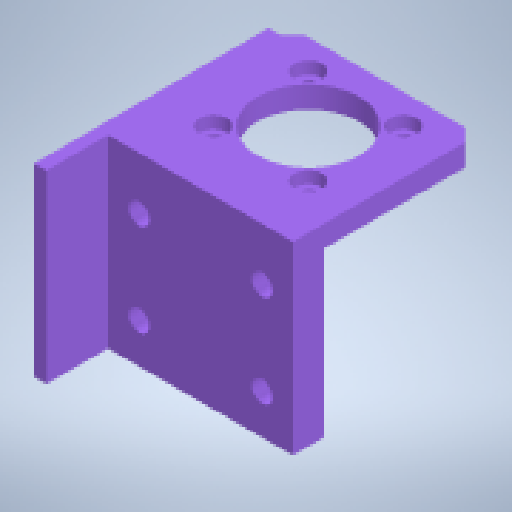
# Autodesk Inventor part: support nema8
Saved by Autodesk Inventor 2025.1 (Build 291241000, 241)
## iProperties
Created: 2025-03-24
Part Number: support nema8
Material: Générique
Document SubType Name: Modeling
Designer: felix
Density: 1 g/cm^3
Appearance: Violet
Author: felix
Autodesk Inventor part; units mm, degrees
ref_plane "YZ Plane" through (0, 0, 0) normal (1, 0, 0) x (0, 1, 0)
ref_plane "XZ Plane" through (0, 0, 0) normal (0, 1, 0) x (-1, 0, 0)
ref_plane "XY Plane" through (0, 0, 0) normal (0, 0, 1) x (1, 0, 0)
sketch "Esquisse1" plane through (0, 0, 0) normal (0, 1, 0) x (-1, 0, 0)
  line L0 (0, 0) -> (30, 0)
  line L1 (30, 0) -> (30, -23)
  line L2 (28, -25) -> (2, -25)
  line L3 (0, -23) -> (0, 0)
  circle A0 centre (15, -12.5) radius 8.25
  line L4 (30, -23) -> (28, -25)
  line L5 (2, -25) -> (0, -23)
  point P0 (0, 0)
  point P1 (30, -25)
  point P2 (0, -25)
  point P3 (11.5, 0)
  point P4 (30, -4)
  point P5 (21, 0)
  point P6 (0, -2)
  point P7 (2, 0)
  dimension "d0" = 25
  dimension "d1" = 30
  dimension "d2" = 16.5
  dimension "d3" = 15
  dimension "d11" = 2
  dimension "d12" = 2
  dimension "d13" = 2
  dimension "d14" = 2
  dimension "d47" = 12.5
  constraints: 13 point on line, 12 end point, 2 parallel, 1 centre point, 1 horizontal, 1 perpendicular
  measures "d0" distance of point (30, 0) point (30, -25)
  measures "d1" distance of point (30, -25) point (0, -25)
  measures "d2" diameter of A0
  measures "d3" distance from line of L3 A0.centre
  measures "d11" distance of L1.end point (30, -25)
  measures "d12" distance of L2.start point (30, -25)
  measures "d13" distance of L2.end point (0, -25)
  measures "d14" distance of L3.start point (0, -25)
  measures "d47" distance from line of L0 A0.centre
extrude "Extrusion1" add sketch "Esquisse1" along normal blind 3.5
sketch "Esquisse2" plane through (0, 3.5, 0) normal (0, 1, 0) x (1, 0, 0)
  circle A0 centre (-15, 12.5) radius 8.25 construction
  circle A1 centre (-15, 12.5) radius 10.8894 construction
  line L0 (-22.7, 4.8) -> (-22.7, 20.2) construction
  line L1 (-22.7, 20.2) -> (-7.3, 20.2) construction
  line L2 (-7.3, 20.2) -> (-7.3, 4.8) construction
  line L3 (-7.3, 4.8) -> (-22.7, 4.8) construction
  point P0 (0, 0)
  dimension "d19" = 15.4
  dimension "d20" = 15.4
  constraints: 8 end point, 5 coincident, 3 point on circle, 2 parallel, 1 centre point, 1 perpendicular, 1 vertical
  measures "d19" distance of L0.start L0.end
  measures "d20" distance of L0.end L1.end
hole "Perçage1" at (-22.7, 3.5, -4.8) at (-22.7, 3.5, -20.2) at (-7.3, 3.5, -20.2) at (-7.3, 3.5, -4.8) direction (0, -1, 0) diameter 2.4 end through all counterbore diameter 4.4 counterbore depth 2 clearance for "Vis d'assemblage à six pans creux" size "M2" standard "Profil M métrique ANSI"
sketch "Esquisse3" plane through (-30, 0, 0) normal (0, 0, 1) x (1, 0, 0)
  line L0 (0, 3.5) -> (30, 3.5) projected
  line L1 (0, 3.5) -> (30, 3.5)
  line L2 (30, 3.5) -> (30, -26.5)
  line L3 (30, -26.5) -> (0, -26.5)
  line L4 (0, -26.5) -> (0, 3.5)
  point P0 (30, 0)
  point P1 (30, 3.5)
  dimension "d29" = 30
  dimension "d48" = 30
  dimension "d49" = 30
  constraints: 8 end point, 2 parallel, 1 horizontal, 1 perpendicular
  measures "d29" distance of L3.end L0.start
  measures "d48" distance of L2.end L3.end
  measures "d49" distance of L0.start L0.end
extrude "Extrusion2" add sketch "Esquisse3" along normal blind 5
sketch "Esquisse4" plane through (-30, 0, -23) normal (-1, 0, 0) x (0, 0, 1)
  line L0 (0, 3.5) -> (28, 3.5) projected
  line L1 (28, 3.5) -> (0, 3.5)
  line L2 (0, 3.5) -> (0, 0)
  line L3 (0, 0) -> (-2, 0) projected
  line L4 (26.5, -26.5) -> (0, 0)
  line L5 (28, 3.5) -> (28, -26.5) projected
  line L6 (28, -26.5) -> (26.5, -26.5)
  line L7 (28, 3.5) -> (38, 3.5)
  line L8 (38, 3.5) -> (38, -26.5)
  line L9 (38, -26.5) -> (21.647, -26.5)
  point P0 (23, 0)
  point P1 (24.5, -21)
  point P2 (0, 3.5)
  point P3 (21, -21)
  dimension "d50" = 30
  dimension "d51" = 30
  dimension "d52" = 10
  constraints: 14 end point, 3 horizontal, 2 perpendicular, 2 point on line, 1 parallel, 1 other
  measures "d50" distance of L0.end L6.start
  measures "d51" distance of L7.end L8.end
  measures "d52" distance of L0.end L7.end
extrude "Extrusion3" add sketch "Esquisse4" along normal blind 2
sketch "Esquisse5" plane through (-30, 0, 0) normal (0, 0, -1) x (-1, 0, 0)
  line L0 (-5, -5) -> (-25, -5) construction
  line L1 (-25, -5) -> (-25, -20) construction
  line L2 (-25, -20) -> (-5, -20) construction
  line L3 (-5, -20) -> (-5, -5) construction
  line L4 (-28, 0) -> (-2, 0) construction
  line L5 (0, 0) -> (0, -23) construction
  point P0 (-30, 0)
  point P1 (0, -21)
  dimension "d36" = 15
  dimension "d37" = 20
  dimension "d38" = 5
  dimension "d39" = 5
  constraints: 8 end point, 4 coincident, 2 parallel, 1 horizontal, 1 perpendicular
  measures "d36" distance of L2.end L0.start
  measures "d37" distance of L1.end L2.end
  measures "d38" distance between parallel lines of L4 L0
  measures "d39" distance between parallel lines of L5 L3
hole "Perçage2" at (-25, -5, 0) at (-25, -20, 0) at (-5, -20, 0) at (-5, -5, 0) direction (0, 0, 1) diameter 3.4 end through all counterbore diameter 6.5 counterbore depth 3 clearance for "Vis d'assemblage à six pans creux" size "M3" standard "Profil M métrique ANSI"
equation "\"d3\" = 0.5 * d1"
equation "\"d11\" = d9"
equation "\"d12\" = d11"
equation "\"d13\" = d9"
equation "\"d14\" = d13"
equation "\"d47\" = 0.5 * d0"
equation "\"d20\" = d19"
equation "\"d48\" = d49"
equation "\"d51\" = d50"
equation "\"d9\" = 2"
